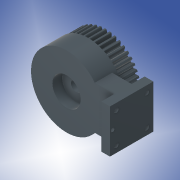
# Autodesk Inventor part: BA013
Saved by Autodesk Inventor 2017 (Build 210142000, 142)
## iProperties
Created: 2017-06-27
Part Number: BA013
Material: ABS Plastic
Document SubType Name: Modeling
Designer: zallen
Density: 1.06 g/cm^3
Appearance: CR Dark Blue
Author: zallen
Autodesk Inventor part; units mm, degrees
ref_plane "YZ Plane" through (0, 0, 0) normal (1, 0, 0) x (0, 1, 0)
ref_plane "XZ Plane" through (0, 0, 0) normal (0, 1, 0) x (-1, 0, 0)
ref_plane "XY Plane" through (0, 0, 0) normal (0, 0, 1) x (1, 0, 0)
sketch "Sketch1" plane through (0, 0, 0) normal (0, 0, 1) x (1, 0, 0)
  circle A0 centre (0, 0) radius 36.25
  circle A1 centre (0, 0) radius 6
  line L0 (0, 0) -> (67.2646, 0) construction
  arc A2 (40.1948, 0.9) -> (36.1948, 2) centre (34.2556, -12.8741) ccw
  arc A3 (36.1948, -2) -> (40.1948, -0.9) centre (34.2556, 12.8741) ccw
  arc A4 (40.1948, -0.9) -> (40.1948, 0.9) centre (20.215, 0) ccw
  arc A5 (36.1948, -2) -> (36.1948, 2) centre (0, 0) ccw
  arc A6 (39.9137, 4.8295) -> (39.6576, 6.6112) centre (20.0093, 2.8769) ccw
  arc A7 (39.6576, 6.6112) -> (35.5417, 7.1307) centre (35.7392, -7.868) ccw
  arc A8 (36.111, 3.1714) -> (39.9137, 4.8295) centre (32.0748, 17.6182) ccw
  circle A9 centre (0, 0) radius 36.25
  arc A10 (38.8202, 10.4606) -> (38.3131, 12.1877) centre (19.3962, 5.6952) ccw
  arc A11 (38.3131, 12.1877) -> (34.1652, 12.1162) centre (36.4951, -2.7017) ccw
  arc A12 (35.2921, 8.2783) -> (38.8202, 10.4606) centre (29.241, 22.0036) ccw
  circle A13 centre (0, 0) radius 36.25
  arc A14 (36.9363, 15.8788) -> (36.1886, 17.5162) centre (18.3883, 8.3976) ccw
  arc A15 (36.1886, 17.5162) -> (32.0931, 16.8551) centre (36.5081, 2.5196) ccw
  arc A16 (33.7548, 13.2166) -> (36.9363, 15.8788) centre (25.8119, 25.941) ccw
  circle A17 centre (0, 0) radius 36.25
  arc A18 (34.3006, 20.9738) -> (33.3274, 22.4881) centre (17.006, 10.9291) ccw
  arc A19 (33.3274, 22.4881) -> (29.3677, 21.2509) centre (35.778, 7.6896) ccw
  arc A20 (31.5303, 17.8859) -> (34.3006, 20.9738) centre (21.8574, 29.3504) ccw
  circle A21 centre (0, 0) radius 36.25
  arc A22 (30.9666, 25.6418) -> (29.7878, 27.0022) centre (15.2775, 13.238) ccw
  arc A23 (29.7878, 27.0022) -> (26.0445, 25.214) centre (34.3195, 12.7031) ccw
  arc A24 (28.6639, 22.191) -> (30.9666, 25.6418) centre (17.4579, 32.1623) ccw
  circle A25 centre (0, 0) radius 36.25
  arc A26 (27.0022, 29.7878) -> (25.6418, 30.9666) centre (13.238, 15.2775) ccw
  arc A27 (25.6418, 30.9666) -> (22.191, 28.6639) centre (32.1623, 17.4579) ccw
  arc A28 (25.214, 26.0445) -> (27.0022, 29.7878) centre (12.7031, 34.3195) ccw
  circle A29 centre (0, 0) radius 36.25
  arc A30 (22.4881, 33.3274) -> (20.9738, 34.3006) centre (10.9291, 17.006) ccw
  arc A31 (20.9738, 34.3006) -> (17.8859, 31.5303) centre (29.3504, 21.8574) ccw
  arc A32 (21.2509, 29.3677) -> (22.4881, 33.3274) centre (7.6896, 35.778) ccw
  circle A33 centre (0, 0) radius 36.25
  arc A34 (17.5162, 36.1886) -> (15.8788, 36.9363) centre (8.3976, 18.3883) ccw
  arc A35 (15.8788, 36.9363) -> (13.2166, 33.7548) centre (25.941, 25.8119) ccw
  arc A36 (16.8551, 32.0931) -> (17.5162, 36.1886) centre (2.5196, 36.5081) ccw
  circle A37 centre (0, 0) radius 36.25
  arc A38 (12.1877, 38.3131) -> (10.4606, 38.8202) centre (5.6952, 19.3962) ccw
  arc A39 (10.4606, 38.8202) -> (8.2783, 35.2921) centre (22.0036, 29.241) ccw
  arc A40 (12.1162, 34.1652) -> (12.1877, 38.3131) centre (-2.7017, 36.4951) ccw
  circle A41 centre (0, 0) radius 36.25
  arc A42 (6.6112, 39.6576) -> (4.8295, 39.9137) centre (2.8769, 20.0093) ccw
  arc A43 (4.8295, 39.9137) -> (3.1714, 36.111) centre (17.6182, 32.0748) ccw
  arc A44 (7.1307, 35.5417) -> (6.6112, 39.6576) centre (-7.868, 35.7392) ccw
  circle A45 centre (0, 0) radius 36.25
  arc A46 (0.9, 40.1948) -> (-0.9, 40.1948) centre (0, 20.215) ccw
  arc A47 (-0.9, 40.1948) -> (-2, 36.1948) centre (12.8741, 34.2556) ccw
  arc A48 (2, 36.1948) -> (0.9, 40.1948) centre (-12.8741, 34.2556) ccw
  circle A49 centre (0, 0) radius 36.25
  arc A50 (-4.8295, 39.9137) -> (-6.6112, 39.6576) centre (-2.8769, 20.0093) ccw
  arc A51 (-6.6112, 39.6576) -> (-7.1307, 35.5417) centre (7.868, 35.7392) ccw
  arc A52 (-3.1714, 36.111) -> (-4.8295, 39.9137) centre (-17.6182, 32.0748) ccw
  circle A53 centre (0, 0) radius 36.25
  arc A54 (-10.4606, 38.8202) -> (-12.1877, 38.3131) centre (-5.6952, 19.3962) ccw
  arc A55 (-12.1877, 38.3131) -> (-12.1162, 34.1652) centre (2.7017, 36.4951) ccw
  arc A56 (-8.2783, 35.2921) -> (-10.4606, 38.8202) centre (-22.0036, 29.241) ccw
  circle A57 centre (0, 0) radius 36.25
  arc A58 (-15.8788, 36.9363) -> (-17.5162, 36.1886) centre (-8.3976, 18.3883) ccw
  arc A59 (-17.5162, 36.1886) -> (-16.8551, 32.0931) centre (-2.5196, 36.5081) ccw
  arc A60 (-13.2166, 33.7548) -> (-15.8788, 36.9363) centre (-25.941, 25.8119) ccw
  circle A61 centre (0, 0) radius 36.25
  arc A62 (-20.9738, 34.3006) -> (-22.4881, 33.3274) centre (-10.9291, 17.006) ccw
  arc A63 (-22.4881, 33.3274) -> (-21.2509, 29.3677) centre (-7.6896, 35.778) ccw
  arc A64 (-17.8859, 31.5303) -> (-20.9738, 34.3006) centre (-29.3504, 21.8574) ccw
  circle A65 centre (0, 0) radius 36.25
  arc A66 (-25.6418, 30.9666) -> (-27.0022, 29.7878) centre (-13.238, 15.2775) ccw
  arc A67 (-27.0022, 29.7878) -> (-25.214, 26.0445) centre (-12.7031, 34.3195) ccw
  arc A68 (-22.191, 28.6639) -> (-25.6418, 30.9666) centre (-32.1623, 17.4579) ccw
  circle A69 centre (0, 0) radius 36.25
  arc A70 (-29.7878, 27.0022) -> (-30.9666, 25.6418) centre (-15.2775, 13.238) ccw
  arc A71 (-30.9666, 25.6418) -> (-28.6639, 22.191) centre (-17.4579, 32.1623) ccw
  arc A72 (-26.0445, 25.214) -> (-29.7878, 27.0022) centre (-34.3195, 12.7031) ccw
  circle A73 centre (0, 0) radius 36.25
  arc A74 (-33.3274, 22.4881) -> (-34.3006, 20.9738) centre (-17.006, 10.9291) ccw
  arc A75 (-34.3006, 20.9738) -> (-31.5303, 17.8859) centre (-21.8574, 29.3504) ccw
  arc A76 (-29.3677, 21.2509) -> (-33.3274, 22.4881) centre (-35.778, 7.6896) ccw
  circle A77 centre (0, 0) radius 36.25
  arc A78 (-36.1886, 17.5162) -> (-36.9363, 15.8788) centre (-18.3883, 8.3976) ccw
  arc A79 (-36.9363, 15.8788) -> (-33.7548, 13.2166) centre (-25.8119, 25.941) ccw
  arc A80 (-32.0931, 16.8551) -> (-36.1886, 17.5162) centre (-36.5081, 2.5196) ccw
  circle A81 centre (0, 0) radius 36.25
  arc A82 (-38.3131, 12.1877) -> (-38.8202, 10.4606) centre (-19.3962, 5.6952) ccw
  arc A83 (-38.8202, 10.4606) -> (-35.2921, 8.2783) centre (-29.241, 22.0036) ccw
  arc A84 (-34.1652, 12.1162) -> (-38.3131, 12.1877) centre (-36.4951, -2.7017) ccw
  circle A85 centre (0, 0) radius 36.25
  arc A86 (-39.6576, 6.6112) -> (-39.9137, 4.8295) centre (-20.0093, 2.8769) ccw
  arc A87 (-39.9137, 4.8295) -> (-36.111, 3.1714) centre (-32.0748, 17.6182) ccw
  arc A88 (-35.5417, 7.1307) -> (-39.6576, 6.6112) centre (-35.7392, -7.868) ccw
  circle A89 centre (0, 0) radius 36.25
  arc A90 (-40.1948, 0.9) -> (-40.1948, -0.9) centre (-20.215, 0) ccw
  arc A91 (-40.1948, -0.9) -> (-36.1948, -2) centre (-34.2556, 12.8741) ccw
  arc A92 (-36.1948, 2) -> (-40.1948, 0.9) centre (-34.2556, -12.8741) ccw
  circle A93 centre (0, 0) radius 36.25
  arc A94 (-39.9137, -4.8295) -> (-39.6576, -6.6112) centre (-20.0093, -2.8769) ccw
  arc A95 (-39.6576, -6.6112) -> (-35.5417, -7.1307) centre (-35.7392, 7.868) ccw
  arc A96 (-36.111, -3.1714) -> (-39.9137, -4.8295) centre (-32.0748, -17.6182) ccw
  circle A97 centre (0, 0) radius 36.25
  arc A98 (-38.8202, -10.4606) -> (-38.3131, -12.1877) centre (-19.3962, -5.6952) ccw
  arc A99 (-38.3131, -12.1877) -> (-34.1652, -12.1162) centre (-36.4951, 2.7017) ccw
  arc A100 (-35.2921, -8.2783) -> (-38.8202, -10.4606) centre (-29.241, -22.0036) ccw
  circle A101 centre (0, 0) radius 36.25
  arc A102 (-36.9363, -15.8788) -> (-36.1886, -17.5162) centre (-18.3883, -8.3976) ccw
  arc A103 (-36.1886, -17.5162) -> (-32.0931, -16.8551) centre (-36.5081, -2.5196) ccw
  arc A104 (-33.7548, -13.2166) -> (-36.9363, -15.8788) centre (-25.8119, -25.941) ccw
  circle A105 centre (0, 0) radius 36.25
  arc A106 (-34.3006, -20.9738) -> (-33.3274, -22.4881) centre (-17.006, -10.9291) ccw
  arc A107 (-33.3274, -22.4881) -> (-29.3677, -21.2509) centre (-35.778, -7.6896) ccw
  arc A108 (-31.5303, -17.8859) -> (-34.3006, -20.9738) centre (-21.8574, -29.3504) ccw
  circle A109 centre (0, 0) radius 36.25
  arc A110 (-30.9666, -25.6418) -> (-29.7878, -27.0022) centre (-15.2775, -13.238) ccw
  arc A111 (-29.7878, -27.0022) -> (-26.0445, -25.214) centre (-34.3195, -12.7031) ccw
  arc A112 (-28.6639, -22.191) -> (-30.9666, -25.6418) centre (-17.4579, -32.1623) ccw
  circle A113 centre (0, 0) radius 36.25
  arc A114 (-27.0022, -29.7878) -> (-25.6418, -30.9666) centre (-13.238, -15.2775) ccw
  arc A115 (-25.6418, -30.9666) -> (-22.191, -28.6639) centre (-32.1623, -17.4579) ccw
  arc A116 (-25.214, -26.0445) -> (-27.0022, -29.7878) centre (-12.7031, -34.3195) ccw
  circle A117 centre (0, 0) radius 36.25
  arc A118 (-22.4881, -33.3274) -> (-20.9738, -34.3006) centre (-10.9291, -17.006) ccw
  arc A119 (-20.9738, -34.3006) -> (-17.8859, -31.5303) centre (-29.3504, -21.8574) ccw
  arc A120 (-21.2509, -29.3677) -> (-22.4881, -33.3274) centre (-7.6896, -35.778) ccw
  circle A121 centre (0, 0) radius 36.25
  arc A122 (-17.5162, -36.1886) -> (-15.8788, -36.9363) centre (-8.3976, -18.3883) ccw
  arc A123 (-15.8788, -36.9363) -> (-13.2166, -33.7548) centre (-25.941, -25.8119) ccw
  arc A124 (-16.8551, -32.0931) -> (-17.5162, -36.1886) centre (-2.5196, -36.5081) ccw
  circle A125 centre (0, 0) radius 36.25
  arc A126 (-12.1877, -38.3131) -> (-10.4606, -38.8202) centre (-5.6952, -19.3962) ccw
  arc A127 (-10.4606, -38.8202) -> (-8.2783, -35.2921) centre (-22.0036, -29.241) ccw
  arc A128 (-12.1162, -34.1652) -> (-12.1877, -38.3131) centre (2.7017, -36.4951) ccw
  circle A129 centre (0, 0) radius 36.25
  arc A130 (-6.6112, -39.6576) -> (-4.8295, -39.9137) centre (-2.8769, -20.0093) ccw
  arc A131 (-4.8295, -39.9137) -> (-3.1714, -36.111) centre (-17.6182, -32.0748) ccw
  arc A132 (-7.1307, -35.5417) -> (-6.6112, -39.6576) centre (7.868, -35.7392) ccw
  circle A133 centre (0, 0) radius 36.25
  arc A134 (-0.9, -40.1948) -> (0.9, -40.1948) centre (0, -20.215) ccw
  arc A135 (0.9, -40.1948) -> (2, -36.1948) centre (-12.8741, -34.2556) ccw
  arc A136 (-2, -36.1948) -> (-0.9, -40.1948) centre (12.8741, -34.2556) ccw
  circle A137 centre (0, 0) radius 36.25
  arc A138 (4.8295, -39.9137) -> (6.6112, -39.6576) centre (2.8769, -20.0093) ccw
  arc A139 (6.6112, -39.6576) -> (7.1307, -35.5417) centre (-7.868, -35.7392) ccw
  arc A140 (3.1714, -36.111) -> (4.8295, -39.9137) centre (17.6182, -32.0748) ccw
  circle A141 centre (0, 0) radius 36.25
  arc A142 (10.4606, -38.8202) -> (12.1877, -38.3131) centre (5.6952, -19.3962) ccw
  arc A143 (12.1877, -38.3131) -> (12.1162, -34.1652) centre (-2.7017, -36.4951) ccw
  arc A144 (8.2783, -35.2921) -> (10.4606, -38.8202) centre (22.0036, -29.241) ccw
  circle A145 centre (0, 0) radius 36.25
  arc A146 (15.8788, -36.9363) -> (17.5162, -36.1886) centre (8.3976, -18.3883) ccw
  arc A147 (17.5162, -36.1886) -> (16.8551, -32.0931) centre (2.5196, -36.5081) ccw
  arc A148 (13.2166, -33.7548) -> (15.8788, -36.9363) centre (25.941, -25.8119) ccw
  circle A149 centre (0, 0) radius 36.25
  arc A150 (20.9738, -34.3006) -> (22.4881, -33.3274) centre (10.9291, -17.006) ccw
  arc A151 (22.4881, -33.3274) -> (21.2509, -29.3677) centre (7.6896, -35.778) ccw
  arc A152 (17.8859, -31.5303) -> (20.9738, -34.3006) centre (29.3504, -21.8574) ccw
  circle A153 centre (0, 0) radius 36.25
  arc A154 (25.6418, -30.9666) -> (27.0022, -29.7878) centre (13.238, -15.2775) ccw
  arc A155 (27.0022, -29.7878) -> (25.214, -26.0445) centre (12.7031, -34.3195) ccw
  arc A156 (22.191, -28.6639) -> (25.6418, -30.9666) centre (32.1623, -17.4579) ccw
  circle A157 centre (0, 0) radius 36.25
  arc A158 (29.7878, -27.0022) -> (30.9666, -25.6418) centre (15.2775, -13.238) ccw
  arc A159 (30.9666, -25.6418) -> (28.6639, -22.191) centre (17.4579, -32.1623) ccw
  arc A160 (26.0445, -25.214) -> (29.7878, -27.0022) centre (34.3195, -12.7031) ccw
  circle A161 centre (0, 0) radius 36.25
  arc A162 (33.3274, -22.4881) -> (34.3006, -20.9738) centre (17.006, -10.9291) ccw
  arc A163 (34.3006, -20.9738) -> (31.5303, -17.8859) centre (21.8574, -29.3504) ccw
  arc A164 (29.3677, -21.2509) -> (33.3274, -22.4881) centre (35.778, -7.6896) ccw
  circle A165 centre (0, 0) radius 36.25
  arc A166 (36.1886, -17.5162) -> (36.9363, -15.8788) centre (18.3883, -8.3976) ccw
  arc A167 (36.9363, -15.8788) -> (33.7548, -13.2166) centre (25.8119, -25.941) ccw
  arc A168 (32.0931, -16.8551) -> (36.1886, -17.5162) centre (36.5081, -2.5196) ccw
  circle A169 centre (0, 0) radius 36.25
  arc A170 (38.3131, -12.1877) -> (38.8202, -10.4606) centre (19.3962, -5.6952) ccw
  arc A171 (38.8202, -10.4606) -> (35.2921, -8.2783) centre (29.241, -22.0036) ccw
  arc A172 (34.1652, -12.1162) -> (38.3131, -12.1877) centre (36.4951, 2.7017) ccw
  circle A173 centre (0, 0) radius 36.25
  arc A174 (39.6576, -6.6112) -> (39.9137, -4.8295) centre (20.0093, -2.8769) ccw
  arc A175 (39.9137, -4.8295) -> (36.111, -3.1714) centre (32.0748, -17.6182) ccw
  arc A176 (35.5417, -7.1307) -> (39.6576, -6.6112) centre (35.7392, 7.868) ccw
  circle A177 centre (0, 0) radius 36.25
  point P0 (40.215, 0)
  point P1 (39.8057, 5.7232)
  point P2 (38.5861, 11.3299)
  point P3 (36.5809, 16.7059)
  point P4 (33.831, 21.7419)
  point P5 (30.3925, 26.3353)
  point P6 (26.3353, 30.3925)
  point P7 (21.7419, 33.831)
  point P8 (16.7059, 36.5809)
  point P9 (11.3299, 38.5861)
  point P10 (5.7232, 39.8057)
  point P11 (0, 40.215)
  point P12 (-5.7232, 39.8057)
  point P13 (-11.3299, 38.5861)
  point P14 (-16.7059, 36.5809)
  point P15 (-21.7419, 33.831)
  point P16 (-26.3353, 30.3925)
  point P17 (-30.3925, 26.3353)
  point P18 (-33.831, 21.7419)
  point P19 (-36.5809, 16.7059)
  point P20 (-38.5861, 11.3299)
  point P21 (-39.8057, 5.7232)
  point P22 (-40.215, 0)
  point P23 (-39.8057, -5.7232)
  point P24 (-38.5861, -11.3299)
  point P25 (-36.5809, -16.7059)
  point P26 (-33.831, -21.7419)
  point P27 (-30.3925, -26.3353)
  point P28 (-26.3353, -30.3925)
  point P29 (-21.7419, -33.831)
  point P30 (-16.7059, -36.5809)
  point P31 (-11.3299, -38.5861)
  point P32 (-5.7232, -39.8057)
  point P33 (0, -40.215)
  point P34 (5.7232, -39.8057)
  point P35 (11.3299, -38.5861)
  point P36 (16.7059, -36.5809)
  point P37 (21.7419, -33.831)
  point P38 (26.3353, -30.3925)
  point P39 (30.3925, -26.3353)
  point P40 (33.831, -21.7419)
  point P41 (36.5809, -16.7059)
  point P42 (38.5861, -11.3299)
  point P43 (39.8057, -5.7232)
  dimension "d0" = 72.5
  dimension "d1" = 12
  dimension "d2" = 15
  dimension "d3" = 15
  dimension "d4" = 20
  dimension "d5" = 4
  dimension "d10" = 2
  dimension "d12" = 1.8
  dimension "d15" = 360
  constraints: 355 point on circle, 178 centre point, 2 coincident, 2 end point, 2 vertical alignment, 1 concentric, 1 horizontal, 1 point on line, 573 other
  measures "d0" diameter of A0
  measures "d1" diameter of A1
  measures "d2" radius of A2
  measures "d3" radius of A3
  measures "d4" radius of A4
  measures "d5" horizontal distance of A2.start A0.start
  measures "d10" distance from line of L0 A0.start
  measures "d12" distance of A3.end A2.start
extrude "Extrusion1" add sketch "Sketch1" along normal blind 20
sketch "Sketch2" plane through (0, 0, 20) normal (0, 0, 1) x (1, 0, 0)
  circle A0 centre (0, 0) radius 6 projected
  circle A1 centre (0, 0) radius 41
  dimension "d19" = 82
  constraints: 1 centre point, 1 coincident
  measures "d19" diameter of A1
extrude "Extrusion2" add sketch "Sketch2" along normal blind 15
sketch "Sketch11" plane through (0, 0, 35) normal (0, 0, 1) x (1, 0, 0)
  circle A0 centre (0, 0) radius 6 projected
  circle A1 centre (0, 0) radius 41
  dimension "d59" = 82
  constraints: 1 centre point, 1 coincident
  measures "d59" diameter of A1
extrude "Extrusion11" add sketch "Sketch11" along normal blind 10
sketch "Sketch12" plane through (0, 0, 45) normal (0, 0, 1) x (1, 0, 0)
  circle A0 centre (0, 0) radius 16.25
  dimension "d62" = 32.5
  constraints: 1 centre point, 1 coincident
  measures "d62" diameter of A0
extrude "Extrusion12" cut sketch "Sketch12" against normal blind 11
sketch "Sketch13" plane through (0, 0, 0) normal (0, 0, -1) x (-1, 0, 0)
  circle A0 centre (0, 0) radius 16.25 projected
extrude "Extrusion13" cut sketch "Sketch13" against normal blind 11
sketch "Sketch14" plane through (0, 0, 45) normal (0, 0, 1) x (1, 0, 0)
  line L0 (0, -25) -> (55, -25)
  line L1 (55, -25) -> (55, 25)
  line L2 (55, 25) -> (0, 25)
  line L3 (0, 25) -> (0, -25)
  circle A0 centre (0, 0) radius 16.25 projected
  circle A1 centre (0, 0) radius 16.25 projected
  arc A2 (0, -16.25) -> (0, 16.25) centre (0, 0) ccw
  dimension "d67" = 55
  dimension "d68" = 50
  constraints: 8 end point, 6 point on circle, 2 midpoint, 2 parallel, 2 point on line, 1 centre point, 1 concentric, 1 horizontal, 1 perpendicular
  measures "d67" distance of L2.end L1.end
  measures "d68" distance of L1.end L0.end
extrude "Extrusion15" add sketch "Sketch14" against normal blind 20 contours L3 A0 L2 L1 L0
sketch "Sketch15" plane through (55, -25, 45) normal (1, 0, 0) x (0, 0, -1)
  line L0 (-15, 0) -> (35, 0)
  line L1 (35, 0) -> (35, 50)
  line L2 (35, 50) -> (-15, 50)
  line L3 (-15, 50) -> (-15, 0)
  line L4 (0, 0) -> (20, 0) projected
  point P0 (45, 25)
  point P1 (10, 0)
  dimension "d73" = 50
  dimension "d74" = 50
  constraints: 8 end point, 2 midpoint, 2 parallel, 1 horizontal, 1 perpendicular
  measures "d73" distance of L2.end L1.end
  measures "d74" distance of L1.end L0.end
extrude "Extrusion16" add sketch "Sketch15" along normal blind 10
sketch "Sketch16" plane through (65, -25, 45) normal (1, 0, 0) x (0, 0, -1)
  line L0 (-7.5, 42.5) -> (27.5, 42.5) construction
  line L1 (27.5, 42.5) -> (27.5, 7.5) construction
  line L2 (27.5, 7.5) -> (-7.5, 7.5) construction
  line L3 (-7.5, 7.5) -> (-7.5, 42.5) construction
  line L4 (10, 46.9203) -> (31.9203, 25) construction
  line L5 (31.9203, 25) -> (10, 3.0797) construction
  line L6 (10, 3.0797) -> (-11.9203, 25) construction
  line L7 (-11.9203, 25) -> (10, 46.9203) construction
  line L8 (10, 46.9203) -> (10, 3.0797) construction
  line L9 (31.9203, 25) -> (-11.9203, 25) construction
  line L10 (10, 46.9203) -> (41, 46.9203) construction
  line L11 (-15, 0) -> (35, 0) construction
  line L12 (35, 0) -> (35, 50) construction
  line L13 (35, 50) -> (-15, 50) construction
  line L14 (-15, 50) -> (-15, 0) construction
  circle A0 centre (-11.9203, 25) radius 2
  circle A1 centre (-7.5, 42.5) radius 2.5
  circle A2 centre (-7.5, 7.5) radius 2.5
  circle A3 centre (27.5, 7.5) radius 2.5
  circle A4 centre (27.5, 42.5) radius 2.5
  point P0 (10, 25)
  point P1 (10, 25)
  point P2 (27.5, 25)
  point P3 (10, 25)
  point P4 (10, 7.5)
  point P5 (10, 0)
  point P6 (-15, 25)
  dimension "d77" = 35
  dimension "d78" = 35
  dimension "d79" = 31
  dimension "d80" = 45
  dimension "d81" = 31
  dimension "d82" = 4
  dimension "d83" = 5
  dimension "d84" = 5
  dimension "d85" = 5
  dimension "d86" = 5
  constraints: 22 end point, 8 midpoint, 5 centre point, 5 coincident, 4 parallel, 2 horizontal, 2 horizontal alignment, 2 perpendicular, 2 vertical alignment, 1 equal length
  measures "d77" distance of L1.end L2.end
  measures "d78" distance of L0.end L1.end
  measures "d79" distance of L4.start L4.end
  measures "d80" angle of L4 L10
  measures "d81" distance of L4.end L5.end
  measures "d82" diameter of A0
  measures "d83" diameter of A1
  measures "d84" diameter of A2
  measures "d85" diameter of A3
  measures "d86" diameter of A4
extrude "Extrusion17" cut sketch "Sketch16" against normal blind 10
body "Solid1"
